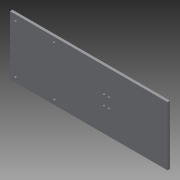
# Autodesk Inventor part: big plate
Saved by Autodesk Inventor 2014 SP1 (Build 180222100, 222)
## iProperties
Created: 2014-02-07
Part Number: big plate
Material: Generic
Document SubType Name: Modeling
Designer: Owner
Density: 1 g/cm^3
Appearance: Default
Author: Owner
Autodesk Inventor part; units mm, degrees
ref_plane "YZ Plane" through (0, 0, 0) normal (1, 0, 0) x (0, 1, 0)
ref_plane "XZ Plane" through (0, 0, 0) normal (0, 1, 0) x (-1, 0, 0)
ref_plane "XY Plane" through (0, 0, 0) normal (0, 0, 1) x (1, 0, 0)
sketch "Sketch1" plane through (0, 0, 0) normal (0, 0, 1) x (1, 0, 0)
  line L0 (-203.2, -76.2) -> (203.2, -76.2)
  line L1 (203.2, -76.2) -> (203.2, 76.2)
  line L2 (203.2, 76.2) -> (-203.2, 76.2)
  line L3 (-203.2, 76.2) -> (-203.2, -76.2)
  line L4 (-203.2, -76.2) -> (203.2, 76.2) construction
  line L5 (203.2, -76.2) -> (-203.2, 76.2) construction
  line L6 (-203.2, 76.2) -> (-189.7296, 62.7296)
  line L7 (-203.2, 76.2) -> (-184.15, 76.2) construction
  line L8 (-203.2, -76.2) -> (-189.7296, -62.7296)
  line L9 (-203.2, -76.2) -> (-184.15, -76.2) construction
  line L10 (-203.2, -76.2) -> (-193.675, -76.2)
  line L11 (-203.2, -76.2) -> (-76.2, -76.2) construction
  line L12 (-76.2, -76.2) -> (-89.6704, -62.7296) construction
  circle A0 centre (-189.7296, 62.7296) radius 3.175
  circle A1 centre (-89.6704, -62.7296) radius 3.175
  circle A2 centre (-189.7296, -62.7296) radius 3.175
  line L13 (-189.7296, 62.7296) -> (-89.6704, -62.7296)
  line L14 (-203.2, 76.2) -> (-76.2, 76.2) construction
  line L15 (-76.2, 76.2) -> (-91.0934, 64.3219) construction
  circle A3 centre (-91.0934, 64.3219) radius 3.175
  point P0 (0, 0)
  dimension "d0" = 406.4
  dimension "d1" = 152.4
  dimension "d2" = 19.05
  dimension "d3" = 45
  dimension "d4" = 19.05
  dimension "d5" = 45
  dimension "d6" = 127
  dimension "d7" = 19.05
  dimension "d8" = 6.35
  dimension "d10" = 6.35
  dimension "d11" = 6.35
  dimension "d15" = 127
  dimension "d16" = 6.35
  constraints: 32 end point, 4 centre point, 4 coincident, 4 perpendicular, 3 horizontal, 3 midpoint, 2 equal length, 2 parallel, 2 point on line
  measures "d0" distance of L2.end L1.end
  measures "d1" distance of L1.end L0.end
  measures "d2" distance of L2.end L6.end
  measures "d3" angle of L6 L7
  measures "d4" distance of L0.start L8.end
  measures "d5" angle of L9 L8
  measures "d6" distance of L0.start L11.end
  measures "d7" distance of L11.end L12.end
  measures "d8" diameter of A0
  measures "d10" diameter of A1
  measures "d11" diameter of A2
  measures "d15" distance of L2.end L14.end
  measures "d16" diameter of A3
extrude "Extrusion2" add sketch "Sketch1" along normal blind 6.35
sketch "Sketch2" plane through (0, 0, 6.35) normal (0, 0, 1) x (1, 0, 0)
  line L0 (203.2, -76.2) -> (203.2, 76.2) projected
  line L1 (-203.2, 76.2) -> (-203.2, -76.2) projected
  line L2 (203.2, 0) -> (38.1, 0) construction
  line L3 (38.1, 0) -> (38.1, 12.7) construction
  line L4 (38.1, 0) -> (38.1, -12.7) construction
  line L5 (38.1, 0) -> (50.8, 0) construction
  line L6 (50.8, 0) -> (50.8, 12.7) construction
  line L7 (50.8, 12.7) -> (50.8, -12.7) construction
  point P0 (0, 0)
  dimension "d19" = 165.1
  dimension "d20" = 12.7
  dimension "d21" = 12.7
  dimension "d22" = 12.7
  dimension "d23" = 12.7
  dimension "d24" = 25.4
  constraints: 12 end point, 4 perpendicular, 1 collinear, 1 midpoint, 1 point on line
  measures "d19" distance of L2.start L2.end
  measures "d20" distance of L2.end L3.end
  measures "d21" distance of L2.end L4.end
  measures "d22" distance of L2.end L5.end
  measures "d23" distance of L5.end L6.end
  measures "d24" distance of L6.end L7.end
hole "Hole1" at (50.8, 12.7, 6.35) at (50.8, -12.7, 6.35) at (38.1, -12.7, 6.35) at (38.1, 12.7, 6.35) direction (0, 0, -1) diameter 6.35 end through all
body "Solid2"
